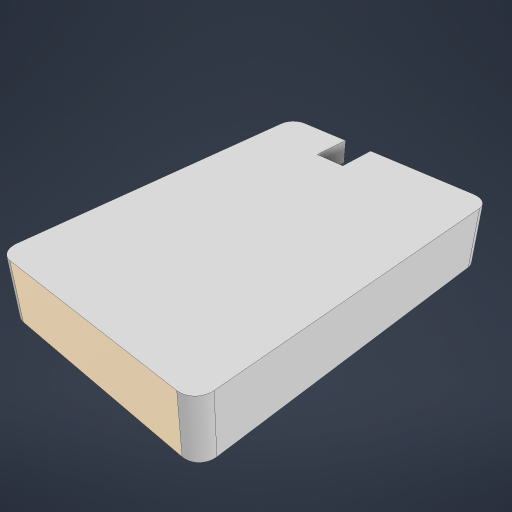
# Autodesk Inventor part: Pieza2
Saved by Autodesk Inventor 2023 (Build 270158000, 158)
## iProperties
Created: 2024-04-13
Part Number: Pieza2
Material: Genérico
Document SubType Name: Modeling
Designer: Diego
Density: 1 g/cm^3
Appearance: Valor por defecto
Author: Diego
Autodesk Inventor part; units mm, degrees
ref_plane "YZ Plane" through (0, 0, 0) normal (1, 0, 0) x (0, 1, 0)
ref_plane "XZ Plane" through (0, 0, 0) normal (0, 1, 0) x (-1, 0, 0)
ref_plane "XY Plane" through (0, 0, 0) normal (0, 0, 1) x (1, 0, 0)
sketch "Boceto1" plane through (0, 0, 0) normal (0, 1, 0) x (-1, 0, 0)
  point P0 (0, 0)
sketch "Boceto2" plane through (0, 0, 0) normal (0, 1, 0) x (-1, 0, 0)
  line L0 (-25, 38) -> (25, 38)
  line L1 (25, 38) -> (25, -38)
  line L2 (25, -38) -> (-25, -38)
  line L3 (-25, -38) -> (-25, 38)
  line L4 (-25, 38) -> (25, -38) construction
  line L5 (25, 38) -> (-25, -38) construction
  line L6 (28, -37) -> (28, 37)
  line L7 (24, 41) -> (-24, 41)
  line L8 (-28, 37) -> (-28, -37)
  line L9 (-24, -41) -> (24, -41)
  arc A0 (28, 37) -> (24, 41) centre (24, 37) ccw
  arc A1 (-24, 41) -> (-28, 37) centre (-24, 37) ccw
  arc A2 (-28, -37) -> (-24, -41) centre (-24, -37) ccw
  arc A3 (24, -41) -> (28, -37) centre (24, -37) ccw
  point P0 (0, 0)
  dimension "d0" = 50
  dimension "d1" = 76
  dimension "d2" = 3
  dimension "d3" = 4
  constraints: 20 end point, 8 point on circle, 8 tangent, 4 centre point, 4 parallel, 3 equal radius, 2 midpoint, 2 perpendicular, 1 horizontal, 3 other
  measures "d0" distance of L1.end L2.end
  measures "d1" distance of L0.end L1.end
  measures "d2" distance between parallel lines of L1 L6
  measures "d3" radius of A0
extrude "Extrusión1" add sketch "Boceto2" along normal blind 14
sketch "Boceto3" plane through (0, 14, 0) normal (0, 1, 0) x (1, 0, 0)
  arc A0 (-28, -37) -> (-24, -41) centre (-24, -37) ccw projected
  line L0 (-24, -41) -> (24, -41) projected
  arc A1 (24, -41) -> (28, -37) centre (24, -37) ccw projected
  line L1 (28, -37) -> (28, 37) projected
  arc A2 (28, 37) -> (24, 41) centre (24, 37) ccw projected
  line L2 (24, 41) -> (-24, 41) projected
  arc A3 (-24, 41) -> (-28, 37) centre (-24, 37) ccw projected
  line L3 (-28, 37) -> (-28, -37) projected
  line L4 (25, -38) -> (-25, -38) projected
  line L5 (-25, -38) -> (-25, 38) projected
  line L6 (-25, 38) -> (25, 38) projected
  line L7 (25, 38) -> (25, -38) projected
  point P0 (0, 0)
extrude "Extrusión2" add sketch "Boceto3" along normal blind 1 contours L3 A3 L2 A2 L1 A1 L0 A0 | L4 L5 L6 L7
sketch "Boceto4" plane through (-25, 0, -38) normal (0, 0, 1) x (1, 0, 0)
  line L0 (0, 0) -> (50, 0) projected
  line L1 (50, 0) -> (50, 14) projected
  line L2 (0, 14) -> (50, 14) projected
  line L3 (0, 0) -> (0, 14) projected
  line L4 (0, 14) -> (10, 14)
  line L5 (10, 14) -> (14, 14)
  line L6 (14, 14) -> (14, 9)
  line L7 (14, 9) -> (10, 9)
  line L8 (10, 9) -> (10, 14)
  line L9 (14, 9) -> (21.5, 9)
  line L10 (21.5, 9) -> (21.5, 14)
  line L11 (21.5, 14) -> (14, 14)
  line L12 (14, 14) -> (14, 9)
  point P0 (25, 0)
  dimension "d8" = 10
  dimension "d9" = 4
  dimension "d10" = 5
  dimension "d11" = 7.5
  dimension "d12" = 5
  constraints: 18 end point, 4 parallel, 2 horizontal, 2 perpendicular, 1 point on line
  measures "d8" distance of L2.start L4.end
  measures "d9" distance of L6.end L7.end
  measures "d10" distance of L5.end L6.end
  measures "d11" distance of L11.end L10.end
  measures "d12" distance of L10.end L9.end
extrude "Extrusión3" cut sketch "Boceto4" against normal through all contours L10 L9 L6 L2
sketch "Boceto5" plane through (-25, 0, -38) normal (0, 0, 1) x (1, 0, 0)
  line L0 (21.5, 14) -> (21.5, 9) projected
  line L1 (21.5, 9) -> (14, 9) projected
  line L2 (14, 9) -> (14, 14) projected
  line L3 (0, 14) -> (14, 14) projected
  line L4 (0, 0) -> (0, 14) projected
  line L5 (0, 0) -> (50, 0) projected
  line L6 (50, 0) -> (50, 14) projected
  line L7 (21.5, 14) -> (50, 14) projected
  line L8 (14, 9) -> (8, 9)
  line L9 (8, 9) -> (8, 14)
  line L10 (8, 14) -> (14, 14)
  line L11 (14, 14) -> (14, 9)
  line L12 (21.5, 14) -> (27.5, 14)
  line L13 (27.5, 14) -> (27.5, 9)
  line L14 (27.5, 9) -> (21.5, 9)
  line L15 (21.5, 9) -> (21.5, 14)
  point P0 (25, 0)
  dimension "d15" = 6
  dimension "d16" = 6
  constraints: 16 end point, 4 parallel, 2 horizontal, 2 perpendicular, 2 point on line
  measures "d15" distance of L9.end L10.end
  measures "d16" distance of L13.end L14.end
extrude "Extrusión4" add sketch "Boceto5" along normal blind 7 contours L7 L13 L14 L0 | L8 L9 L3 L2
sketch "Boceto6" plane through (0, 14, 0) normal (0, -1, 0) x (1, 0, 0)
  line L0 (-3.5, -41) -> (-3.5, -31) projected
  line L1 (-3.5, -31) -> (2.5, -31) projected
  line L2 (2.5, -31) -> (2.5, -38) projected
  line L3 (2.5, -38) -> (25, -38) projected
  line L4 (25, -38) -> (25, 38) projected
  line L5 (25, 38) -> (-25, 38) projected
  line L6 (-25, 38) -> (-25, -38) projected
  line L7 (-25, -38) -> (-17, -38) projected
  line L8 (-17, -38) -> (-17, -31) projected
  line L9 (-17, -31) -> (-11, -31) projected
  line L10 (-11, -31) -> (-11, -41) projected
  line L11 (-3.5, -41) -> (-11, -41) projected
  line L12 (-3.5, -31) -> (-11, -31)
  point P0 (0, 0)
  constraints: 2 end point, 1 horizontal
extrude "Extrusión5" cut sketch "Boceto6" against normal blind 7 contours L11 L10 L12 L0
sketch "Boceto7" plane through (-3.5, 9, -38) normal (0, -1, 0) x (1, 0, 0)
  line L0 (-7.5, 0) -> (-13.5, 0) projected
  line L1 (-7.5, 0) -> (-7.5, 7) projected
  line L2 (-13.5, 7) -> (-7.5, 7) projected
  line L3 (-13.5, 0) -> (-13.5, 7) projected
  line L4 (6, 0) -> (0, 0) projected
  line L5 (6, 0) -> (6, 7) projected
  line L6 (0, 7) -> (6, 7) projected
  line L7 (0, 0) -> (0, 7) projected
  circle A0 centre (-11.25, 3) radius 0.75
  circle A1 centre (3.75, 3) radius 0.75
  point P0 (3.5, 38)
  dimension "d21" = 1.5
  dimension "d22" = 1.5
  dimension "d23" = 15
  dimension "d24" = 2.25
  dimension "d25" = 2.25
  dimension "d30" = 4
  dimension "d31" = 3
  dimension "d32" = 3
  dimension "d33" = 4
  constraints: 2 centre point
  measures "d21" diameter of A0
  measures "d22" diameter of A1
  measures "d23" distance of A0.centre A1.centre
  measures "d24" distance from line of L5 A1.centre
  measures "d25" distance from line of L3 A0.centre
  measures "d30" distance from line of L2 A0.centre
  measures "d31" distance from line of L0 A0.centre
  measures "d32" distance from line of L4 A1.centre
  measures "d33" distance from line of L6 A1.centre
extrude "Extrusión6" cut sketch "Boceto7" against normal blind 3 contours A0 | A1
sketch "Boceto8" plane through (-25, 0, -31) normal (0, 0, 1) x (1, 0, 0)
  line L0 (14, 9) -> (14, 14) projected
  line L1 (8, 14) -> (14, 14) projected
  line L2 (8, 14) -> (8, 9) projected
  line L3 (8, 9) -> (14, 9) projected
  line L4 (27.5, 9) -> (27.5, 14) projected
  line L5 (21.5, 14) -> (27.5, 14) projected
  line L6 (21.5, 14) -> (21.5, 9) projected
  line L7 (21.5, 9) -> (27.5, 9) projected
  line L8 (14, 9) -> (8, 9) projected
  line L9 (14, 9) -> (21.5, 9)
  line L10 (21.5, 9) -> (21.5, 14)
  line L11 (21.5, 14) -> (14, 14)
  line L12 (14, 14) -> (14, 9)
  point P0 (25, 0)
  constraints: 8 end point, 2 parallel, 1 horizontal, 1 perpendicular
extrude "Extrusión7" add sketch "Boceto8" along normal mid plane 1
